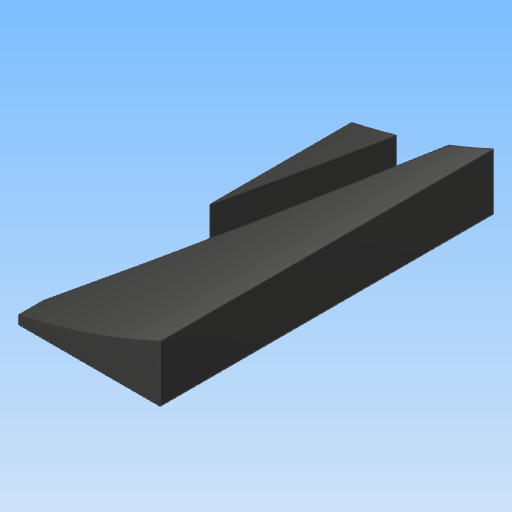
# Autodesk Inventor part: WireGuideToSail1
Saved by Autodesk Inventor 2017 (Build 210142000, 142)
## iProperties
Created: 2018-03-28
Part Number: WireGuideToSail1
Material: ABS Plastic
Document SubType Name: Modeling
Designer: Derek Wider
Density: 1.06 g/cm^3
Appearance: Smooth - Black
Author: Derek Wider
Autodesk Inventor part; units mm, degrees
ref_plane "YZ Plane" through (0, 0, 0) normal (1, 0, 0) x (0, 1, 0)
sketch "Sketch1" plane through (0, 0, 0) normal (0, 0, 1) x (1, 0, 0)
  line L0 (0, 3.175) -> (0, 0)
  line L1 (0, 0) -> (10.795, 0)
  line L2 (10.795, 0) -> (10.795, 6.831)
  arc A0 (0, 3.175) -> (10.795, 6.831) centre (-10.795, 52.8148) ccw
  line L3 (0, 3.175) -> (-10.795, 3.175) construction
  line L4 (-10.795, 3.175) -> (-10.795, 2.0148) construction
  arc A1 (-10.795, 2.0148) -> (0, 3.175) centre (-10.795, 52.8148) ccw construction
  dimension "d0" = 50.8
  dimension "d1" = 3.175
  dimension "d4" = 10.795
  dimension "d11" = 10.795
  constraints: 10 end point, 4 point on circle, 2 centre point, 2 perpendicular, 2 vertical, 1 coincident, 1 concentric, 1 horizontal, 1 line through centre
  measures "d0" radius of A0
  measures "d1" distance of L0.start L0.end
  measures "d4" distance of L0.end L1.end
  measures "d11" distance of L0.start L3.end
extrude "Extrusion1" add sketch "Sketch1" along normal blind 25.4
ref_plane "Work Plane1" through (0, 3.175, 0) normal (0, -1, 0) x (1, 0, 0)
sketch "Sketch2" plane through (0, 3.175, 0) normal (0, -1, 0) x (1, 0, 0)
  line L0 (0, 0) -> (0, 25.4) projected
  line L1 (0, 17.145) -> (5.3975, 0)
  line L2 (10.795, 0) -> (0, 0) projected
  line L3 (0, 25.4) -> (10.795, 25.4) projected
  dimension "d6" = 8.255
  constraints: 2 end point, 1 midpoint, 1 point on line
  measures "d6" distance from line of L3 L1.start
ref_plane "Work Plane2" through (0, 3.175, 17.145) normal (0.3003, 0, -0.9538) x (0, 1, 0)
sketch "Sketch3" plane through (0, 3.175, 17.145) normal (0.3003, 0, -0.9538) x (0, 1, 0)
  line L0 (2.2225, -1.905) -> (-2.2225, -1.905)
  line L1 (-2.2225, -1.905) -> (-2.2225, 1.905)
  line L2 (-2.2225, 1.905) -> (2.2225, 1.905)
  line L3 (2.2225, 1.905) -> (2.2225, -1.905)
  point P0 (-3.175, -5.1484)
  point P1 (0, 0)
  point P2 (2.2225, 0)
  point P3 (0, 1.905)
  dimension "d7" = 4.445
  dimension "d10" = 3.81
  constraints: 8 end point, 2 midpoint, 2 parallel, 1 horizontal, 1 horizontal alignment, 1 perpendicular, 1 vertical alignment
  measures "d7" distance of L0.start L0.end
  measures "d10" distance of L0.end L1.end
extrude "Extrusion2" cut sketch "Sketch3" along normal through all both and the other way through all
chamfer "Chamfer1" distance 2.54 angle 45 1 edges at (10.795, 0, 12.7)
chamfer "Chamfer2" distance 2.54 angle 45 1 edges at (4.1275, 0, 25.4)
body "Solid1"
